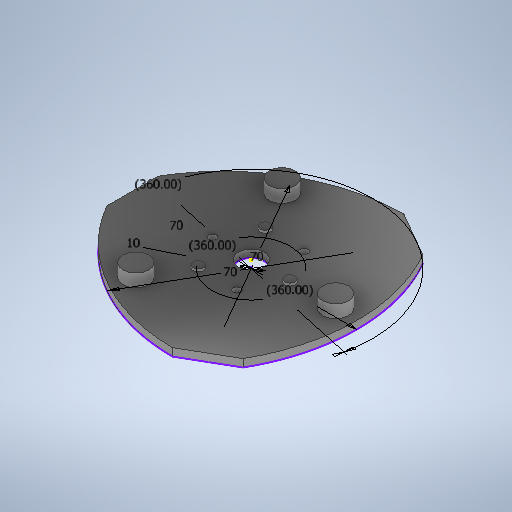
# Autodesk Inventor part: Tool_1
Saved by Autodesk Inventor 2025 (Build 290162000, 162)
## iProperties
Created: 2026-05-15
Part Number: Tool_1
Material: Generic
Document SubType Name: Sheet Metal
Designer: MSI
Density: 1 g/cm^3
Sheet Metal Rule: Default_mm
Appearance: Chrome - Polished Black
Author: MSI
Autodesk Inventor part; units mm, degrees
ref_plane "YZ Plane" through (0, 0, 0) normal (1, 0, 0) x (0, 1, 0)
ref_plane "XZ Plane" through (0, 0, 0) normal (0, 1, 0) x (-1, 0, 0)
ref_plane "XY Plane" through (0, 0, 0) normal (0, 0, 1) x (1, 0, 0)
sketch "Sketch1" plane through (0, 0, 0) normal (0, 1, 0) x (-1, 0, 0)
  circle A0 centre (0, 0) radius 25
  circle A1 centre (0, 0) radius 5
  circle A2 centre (15, 0) radius 1.505
  line L0 (46, 0) -> (46, -10)
  line L1 (46, -10) -> (40, -10)
  line L2 (34, 0) -> (34, -10)
  line L3 (34, -10) -> (40, -10)
  line L4 (34, 0) -> (46, 0)
  line L5 (46, 0) -> (46, 10)
  line L6 (46, 10) -> (34, 10)
  line L7 (34, 10) -> (34, 0)
  line L8 (-23, 39.8372) -> (-14.3397, 44.8372)
  line L9 (-14.3397, 44.8372) -> (-11.3397, 39.641)
  line L10 (-17, 29.4449) -> (-8.3397, 34.4449)
  line L11 (-8.3397, 34.4449) -> (-11.3397, 39.641)
  line L12 (-17, 29.4449) -> (-23, 39.8372)
  line L13 (-23, 39.8372) -> (-31.6603, 34.8372)
  line L14 (-31.6603, 34.8372) -> (-25.6603, 24.4449)
  line L15 (-25.6603, 24.4449) -> (-17, 29.4449)
  line L16 (-23, -39.8372) -> (-31.6603, -34.8372)
  line L17 (-31.6603, -34.8372) -> (-28.6603, -29.641)
  line L18 (-17, -29.4449) -> (-25.6603, -24.4449)
  line L19 (-25.6603, -24.4449) -> (-28.6603, -29.641)
  line L20 (-17, -29.4449) -> (-23, -39.8372)
  line L21 (-23, -39.8372) -> (-14.3397, -44.8372)
  line L22 (-14.3397, -44.8372) -> (-8.3397, -34.4449)
  line L23 (-8.3397, -34.4449) -> (-17, -29.4449)
  circle A3 centre (-7.5, 12.9904) radius 1.505
  circle A4 centre (-7.5, -12.9904) radius 1.505
  circle A5 centre (-15, 0) radius 2.005
  circle A6 centre (7.5, -12.9904) radius 2.005
  circle A7 centre (7.5, 12.9904) radius 2.005
  arc A8 (46, 10) -> (-14.3397, 44.8372) centre (-14.5276, -25.1626) ccw
  arc A9 (-14.3397, -44.8372) -> (46, -10) centre (-14.5276, 25.1626) ccw
  arc A10 (-31.6603, 34.8372) -> (-31.6603, -34.8372) centre (29.0552, 0) ccw
  point P0 (40, 0)
  dimension "d22" = 360
  dimension "d26" = 360
  dimension "d32" = 360
  dimension "d34" = 70
  dimension "d35" = 70
  dimension "d36" = 70
  dimension "d90" = 10
  constraints: 48 end point, 11 centre point, 6 point on circle, 3 coincident, 3 point on line, 2 parallel, 1 horizontal, 1 midpoint, 1 perpendicular, 67 other
  measures "d34" radius of A8
  measures "d35" radius of A9
  measures "d36" radius of A10
  measures "d90" diameter of A1
extrude "Extrusion1" add sketch "Sketch1" along normal blind 3 contours L0 L1 L3 L2 L4 | L4 L7 L6 L5 | A9 L22 L23 L18 L19 L17 A10 L14 L15 L10 L11 L9 A8 L6 L7 L2 L3 L1 | L21 L20 L23 L22 | L9 L11 L10 L12 L8 | L16 L17 L19 L18 L20 | L12 L15 L14 L13
sketch "Sketch2" plane through (0, 3, 0) normal (0, 1, 0) x (1, 0, 0)
  circle A0 centre (32.7082, 0) radius 5
  circle A1 centre (-16.3541, 28.3261) radius 5
  circle A2 centre (-16.3541, -28.3261) radius 5
  point P0 (0, 0)
  dimension "d43" = 10
  dimension "d46" = 360
  constraints: 3 centre point, 7 other
  measures "d43" diameter of A0
extrude "Extrusion4" add sketch "Sketch2" along normal blind 5
extrude "Extrusion7" add sketch "Sketch1" along normal blind 3 contours A0
sketch "Sketch8" plane through (0, 3, 0) normal (0, 1, 0) x (1, 0, 0)
  point P0 (0, 0)
extrude "Extrusion9" add sketch "Sketch1" along normal blind 4 contours A5 | A6 | A7
equation "\"BendRadius\" = Thickness"
equation "\"BendReliefWidth\" = Thickness"
equation "\"BendReliefDepth\" = 0.5 * Thickness"
equation "\"CornerReliefSize\" = 4 * Thickness"
equation "\"MinimumRemnant\" = 2 * Thickness"
equation "\"TransitionRadius\" = BendRadius"
equation "\"JacobiRadiusSize\" = BendRadius"
equation "\"GapSize\" = Thickness"
equation "\"Thickness\" = 0.5"
body "Solid1"
